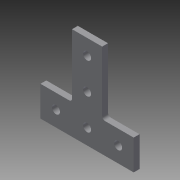
# Autodesk Inventor part: 4080
Saved by Autodesk Inventor 2014 SP2 (Build 180246200, 246)
## iProperties
Created: 2019-11-07
Part Number: 4080
Material: Generic
Catalog Web Link: www.cadenas.de
Description: 4080, 4480, 4080-Black, 4480-Black-Joining Plates - 5 Hole "T" Joining Plate
Vendor: 8020
Document SubType Name: Modeling
Designer: psadmin
Manufacturer: 8020
Mass: 14.244 g
Surface Area: 79.0115 cm^2
Volume: 14.244 cm^3
Density: 1 g/cm^3
Appearance: PSOLRGB-191-191-191
Category: PARTsolutions
Company: 8020
Title: 4080
Author: Cadenas PARTsolutions
Comments: Joining Plates - 5 Hole "T" Joining Plate
PSOL_IDENT_0: {$CADENAS_DATA\23d-libs\8020\inch\joining_plates\4080.prj},176 {VTYP=3D},{NB=4080},{LINA=4080},{NN=4
PSOL_IDENT_1: 080, 4480, 4080-Black, 4480-Black},{DATE=01.10.2019 06:04:23},{GEOMDATE=19.07.2017 16:11:47},{VERSIO
PSOL_IDENT_2: N=},{LINEID=10},{WBVAR=},{WBNUMERIC=}  {NB=4080},{LINA=4080},{KT=DUMMY},{PN=4080},{A=0.500},{B=1.000
PSOL_IDENT_3: },{C=0.970},{D=0.970},{E=3.0000},{F=0.257},{G=0.094},{T=0.188},{W=.096},{COLOR=.75,.75,.75}
NN: 4080, 4480, 4080-Black, 4480-Black
NT: Joining Plates - 5 Hole "T" Joining Plate
NB: 4080
NBSYN: $PN.
LINA: 4080
PN: 4080
A: 0.5
B: 1
C: 0.97
D: 0.97
E: 3
F: 0.257
G: 0.094
T: 0.188
W: .096
SUPPLIER: 8020
ARTICLENO: 4080
BOMINFO: 4080
CREATOR: CADENAS GmbH
Autodesk Inventor part; units mm, degrees
ref_plane "YZ Plane" through (0, 0, 0) normal (1, 0, 0) x (0, 1, 0)
ref_plane "XZ Plane" through (0, 0, 0) normal (0, 1, 0) x (-1, 0, 0)
ref_plane "XY Plane" through (0, 0, 0) normal (0, 0, 1) x (1, 0, 0)
sketch "Sketch_1" plane through (0, 0, 0) normal (0, 0, 1) x (1, 0, 0)
  line L0 (-38.1, 24.638) -> (-38.1, 0)
  line L1 (-38.1, 0) -> (38.1, 0)
  line L2 (38.1, 0) -> (38.1, 24.638)
  line L3 (38.1, 24.638) -> (14.7066, 24.638)
  arc A0 (12.319, 27.0256) -> (14.7066, 24.638) centre (14.7066, 27.0256) ccw
  line L4 (12.319, 27.0256) -> (12.319, 76.2)
  line L5 (12.319, 76.2) -> (-12.319, 76.2)
  line L6 (-12.319, 76.2) -> (-12.319, 27.0256)
  arc A1 (-14.7066, 24.638) -> (-12.319, 27.0256) centre (-14.7066, 27.0256) ccw
  line L7 (-14.7066, 24.638) -> (-38.1, 24.638)
  circle A2 centre (25.4, 12.7) radius 3.2639
  circle A3 centre (0, 12.7) radius 3.2639
  circle A4 centre (0, 63.5) radius 3.2639
  circle A5 centre (0, 38.1) radius 3.2639
  circle A6 centre (-25.4, 12.7) radius 3.2639
  constraints: 16 end point, 7 centre point, 4 point on circle
extrude "Extrusion1" add sketch "Sketch_1" along normal blind 4.7752
body "Solid1"
